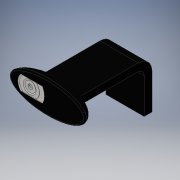
# Autodesk Inventor part: Camera
Saved by Autodesk Inventor 2016 (Build 200138000, 138)
## iProperties
Created: 2015-09-18
Part Number: Camera
Material: Generic
Document SubType Name: Modeling
Designer: lachesis
Density: 1 g/cm^3
Appearance: Default
Author: lachesis
Autodesk Inventor part; units mm, degrees
ref_plane "YZ Plane" through (0, 0, 0) normal (1, 0, 0) x (0, 1, 0)
ref_plane "XZ Plane" through (0, 0, 0) normal (0, 1, 0) x (-1, 0, 0)
ref_plane "XY Plane" through (0, 0, 0) normal (0, 0, 1) x (1, 0, 0)
sketch "Sketch1" plane through (0, 0, 0) normal (0, 0, 1) x (1, 0, 0)
  ellipse E0 centre (0, 0) end of major axis (35.052, 0) minor radius 14.859 (35.052, 0) -> (-35.052, 0) ccw
  line L0 (35.052, 0) -> (-35.052, 0)
  dimension "d0" = 14.859
  dimension "d1" = 35.052
  constraints: 2 end point, 1 coincident, 1 horizontal, 1 horizontal alignment, 4 other
revolve "Revolution1" add sketch "Sketch1" angle 180 about axis through (35.052, 0, 0) along (-1, 0, 0)
ref_plane "Work Plane1" through (0, 0, -10.16) normal (0, 0, 1) x (1, 0, 0)
sketch "Sketch2" plane through (0, 0, -10.16) normal (0, 0, 1) x (1, 0, 0)
  line L0 (17.653, 3.429) -> (-17.653, 3.429)
  line L1 (-17.653, 3.429) -> (-17.653, -3.429)
  line L2 (-17.653, -3.429) -> (17.653, -3.429)
  line L3 (17.653, -3.429) -> (17.653, 3.429)
  point P0 (0, 0)
  point P1 (0, 3.429)
  point P2 (17.653, 0)
  dimension "d4" = 35.306
  dimension "d5" = 6.858
  constraints: 8 end point, 2 midpoint, 2 parallel, 1 horizontal, 1 horizontal alignment, 1 perpendicular, 1 vertical alignment
  measures "d4" distance of L0.start L0.end
  measures "d5" distance of L0.end L1.end
extrude "Extrusion1" add sketch "Sketch2" against normal blind 68.707
sketch "Sketch3" plane through (0, 0, -78.867) normal (0, 0, -1) x (-1, 0, 0)
  line L0 (17.653, 3.429) -> (-17.653, 3.429) projected
  line L1 (-17.653, 3.429) -> (-17.653, -3.429) projected
  line L2 (-17.653, -3.429) -> (17.653, -3.429) projected
  line L3 (17.653, -3.429) -> (17.653, 3.429) projected
  line L4 (17.653, 3.429) -> (-17.653, 3.429) projected
  line L5 (-17.653, 3.429) -> (17.653, 3.429)
  line L6 (17.653, 3.429) -> (17.653, -42.037)
  line L7 (17.653, -42.037) -> (-17.653, -42.037)
  line L8 (-17.653, -42.037) -> (-17.653, 3.429)
  point P0 (0, 0)
  dimension "d8" = 45.466
  constraints: 8 end point, 2 parallel, 1 horizontal, 1 perpendicular
  measures "d8" distance of L0.start L6.end
extrude "Extrusion2" add sketch "Sketch3" against normal blind 7.239 contours L6 L7 L8 L2
sketch "Sketch4" plane through (-17.653, -3.429, -71.628) normal (0, -1, 0) x (1, 0, 0)
  line L0 (27.559, 49.784) -> (7.747, 49.784)
  line L1 (7.747, 49.784) -> (7.747, 47.244)
  line L2 (7.747, 47.244) -> (27.559, 47.244)
  line L3 (27.559, 47.244) -> (27.559, 49.784)
  line L4 (0, 0) -> (35.306, 0) projected
  point P0 (17.653, 71.628)
  point P1 (17.653, 47.244)
  point P2 (17.653, 0)
  dimension "d11" = 47.244
  dimension "d12" = 2.54
  dimension "d13" = 19.812
  constraints: 8 end point, 2 midpoint, 2 parallel, 1 horizontal, 1 perpendicular, 1 vertical alignment
  measures "d11" distance between parallel lines of L2 L4
  measures "d12" distance of L0.end L1.end
  measures "d13" distance of L0.start L0.end
extrude "Extrusion3" add sketch "Sketch4" along normal blind 9.906
fillet "Fillet1" radius 6.35 1 edges at (0, -3.429, -71.628)
fillet "Fillet2" radius 1.27 1 edges at (0, -3.429, -24.384)
sketch "Sketch5" plane through (0, 0, 0) normal (0, 0, 1) x (1, 0, 0)
  line L0 (-29.21, 6.858) -> (29.21, 6.858)
  line L1 (29.21, -6.858) -> (-29.21, -6.858)
  circle A0 centre (-16.51, 0) radius 2.159
  circle A1 centre (-16.51, 0) radius 4.826
  arc A2 (-4.3392, -6.858) -> (-4.3392, 6.858) centre (-16.51, 0) ccw
  arc A3 (-28.6808, 6.858) -> (-29.21, 5.8199) centre (-16.51, 0) ccw
  arc A4 (-29.21, -5.8199) -> (-28.6808, -6.858) centre (-16.51, 0) ccw
  arc A5 (-22.7485, 6.858) -> (-22.7485, -6.858) centre (-16.51, 0) ccw
  arc A6 (-10.2715, -6.858) -> (-10.2715, 6.858) centre (-16.51, 0) ccw
  line L2 (-29.21, -6.858) -> (-29.21, -5.8199)
  line L3 (-29.21, 5.8199) -> (-29.21, 6.858)
  point P0 (0, 0)
  point P1 (29.21, 0)
  point P2 (0, 6.858)
  dimension "d19" = 4.318
  dimension "d20" = 9.652
  dimension "d25" = 13.97
  dimension "d26" = 13.97
  dimension "d27" = 13.97
  dimension "d28" = 9.271
  dimension "d29" = 9.271
  dimension "d45" = 13.716
  dimension "d46" = 58.42
  dimension "d47" = 12.7
  dimension "d48" = 6.858
  dimension "d49" = 90
  dimension "d50" = 29.21
  dimension "d51" = 58.42
  constraints: 10 point on circle, 8 end point, 8 point on line, 7 centre point, 3 coincident, 2 horizontal alignment, 2 parallel, 1 horizontal, 1 midpoint, 1 vertical, 1 vertical alignment
  measures "d19" diameter of A0
  measures "d20" diameter of A1
  measures "d25" radius of A3
  measures "d26" radius of A2
  measures "d27" radius of A4
  measures "d28" radius of A5
  measures "d29" radius of A6
  measures "d45" distance between parallel lines of L1 L0
  measures "d46" distance of L1.start L1.end
  measures "d47" horizontal distance of L1.end A0.centre
  measures "d48" distance from line of L0 point (0, 0)
  measures "d49" angle of L3 L0
  measures "d50" distance from line of point (0, 0) L2
  measures "d51" distance from line of point (29.21, 0) L3
extrude "Extrusion4" cut sketch "Sketch5" against normal blind 0.254 contours L0 A2 L1 A6
extrude "Extrusion5" cut sketch "Sketch5" against normal blind 0.508 contours L0 A6 L1 A5
extrude "Extrusion6" cut sketch "Sketch5" against normal blind 1.016 contours A1
extrude "Extrusion7" cut sketch "Sketch5" against normal blind 2.032 contours A0
draft "FaceDraft1" angle 65 pull direction (0, 0, 1) faces at (-7.5938, 2.5403, -0.4233) fixed edges at (-7.239, 0, -0.254)
draft "FaceDraft2" angle 65 pull direction (0, 0, 1) faces at (-23.2722, 6.3422, -0.1693) fixed edges at (-25.781, 0, -0.508)
draft "FaceDraft3" angle 65 pull direction (0, 0, 1) faces at (-11.6996, -0.3883, -0.8467) fixed edges at (-21.336, 0, -1.016)
draft "FaceDraft4" angle 35 pull direction (0, 0, 1) faces at (-14.358, -0.1737, -1.6933) fixed edges at (-18.669, 0, -1.016)
fillet "Fillet3" radius 1.27 2 edges at (0, -14.859, 0) (0, 14.859, 0)
fillet "Fillet4" radius 12.7 1 edges at (0, 3.429, -78.867)
body "Solid1"
